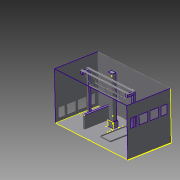
# Autodesk Inventor part: WTC
Saved by Autodesk Inventor 2013 (Build 170138000, 138)
## iProperties
Created: 2010-06-16
Part Number: WTC
Document SubType Name: Modeling
Designer: taylorm
Density: 1 g/cm^3
Material: Generic
Author: taylorm
Autodesk Inventor part; units mm, degrees
(part 1 of 2)
sketch "Sketch2" plane through (0, 0, 0) normal (0, 0, 1) x (1, 0, 0)
  line L0 (-3223.2861, 2012.2183) -> (3796.7139, 2012.2183)
  line L1 (3796.7139, 2012.2183) -> (3796.7139, -1587.7817)
  line L2 (3796.7139, -1587.7817) -> (-3223.2861, -1587.7817)
  line L3 (-3223.2861, -1587.7817) -> (-3223.2861, 2012.2183)
  point P0 (0, 0)
  dimension "d0" = 3600
  dimension "d1" = 7020
  constraints: 8 end point, 2 perpendicular, 1 horizontal, 1 parallel
  measures "d0" distance between parallel lines of L0 L2
  measures "d1" distance between parallel lines of L1 L3
ref_plane "Work Plane1" through (3796.7139, -1587.7817, 0) normal (0, 1, 0) x (-1, 0, 0)
sketch "Sketch4" plane through (3796.7139, -1587.7817, 0) normal (0, 1, 0) x (-1, 0, 0)
  line L0 (0, 0) -> (7020, 0) projected
  line L1 (0, 0) -> (0, -3820)
  line L2 (0, -3820) -> (7020, -3820)
  line L3 (7020, -3820) -> (7020, 0)
  point P0 (3796.7139, 0)
  dimension "d3" = 3820
  constraints: 6 end point, 3 perpendicular
  measures "d3" distance between parallel lines of L0 L2
ref_plane "Work Plane3" through (3796.7139, 2012.2183, 0) normal (0, 1, 0) x (-1, 0, 0)
sketch "Sketch5" plane through (3796.7139, 2012.2183, 0) normal (0, 1, 0) x (-1, 0, 0)
  line L0 (7020, -3820) -> (7020, 0) projected
  line L1 (0, -3820) -> (7020, -3820) projected
  line L2 (0, 0) -> (0, -3820) projected
  line L3 (7020, 0) -> (7020, -3820)
  line L4 (0, -3820) -> (0, 0)
  line L5 (0, -3820) -> (7020, -3820)
  point P0 (3796.7139, 0)
  constraints: 6 end point, 3 collinear
ref_plane "Work Plane4" through (3796.7139, 2012.2183, 0) normal (-1, 0, 0) x (0, 0, -1)
sketch "Sketch6" plane through (3796.7139, 2012.2183, 0) normal (-1, 0, 0) x (0, 0, -1)
  line L0 (0, 0) -> (3820, 0) projected
  line L1 (0, 3600) -> (3820, 3600) projected
  line L2 (0, 0) -> (0, 3600) projected
  line L3 (3820, 0) -> (3820, 3600)
  point P0 (0, 2012.2183)
  constraints: 2 end point, 1 parallel
ref_plane "Work Plane5" through (-3223.2861, -1587.7817, 0) normal (1, 0, 0) x (0, 0, -1)
sketch "Sketch7" plane through (-3223.2861, -1587.7817, 0) normal (1, 0, 0) x (0, 0, -1)
  line L0 (3820, 3600) -> (3820, 0) projected
  line L1 (3820, 0) -> (3820, 3600)
  point P0 (0, 1587.7817)
  constraints: 2 end point, 1 collinear
sketch "Sketch8" plane through (0, 0, 0) normal (0, 0, 1) x (1, 0, 0)
  line L0 (-663.2861, -147.7817) -> (-663.2861, -547.7817)
  line L1 (-663.2861, -547.7817) -> (-143.2861, -547.7817)
  line L2 (-143.2861, -547.7817) -> (-143.2861, -147.7817)
  line L3 (-143.2861, -147.7817) -> (-663.2861, -147.7817)
  line L4 (-3223.2861, -1587.7817) -> (-3223.2861, 2012.2183) projected
  line L5 (-3223.2861, 2012.2183) -> (3796.7139, 2012.2183) projected
  point P0 (0, 0)
  dimension "d4" = 2160
  dimension "d5" = 2560
  dimension "d6" = 400
  dimension "d7" = 520
  constraints: 8 end point, 2 parallel, 2 perpendicular, 1 vertical
  measures "d4" distance between parallel lines of L5 L3
  measures "d5" distance between parallel lines of L0 L4
  measures "d6" distance between parallel lines of L1 L3
  measures "d7" distance between parallel lines of L2 L0
ref_plane "Work Plane6" through (-663.2861, -147.7817, 0) normal (0, 1, 0) x (-1, 0, 0)
sketch "Sketch9" plane through (-663.2861, -147.7817, 0) normal (0, 1, 0) x (-1, 0, 0)
  line L0 (-520, 0) -> (0, 0) projected
  line L1 (0, 0) -> (0, -460)
  line L2 (0, -460) -> (-520, -460)
  line L3 (-520, -460) -> (-520, 0)
  point P0 (-663.2861, 0)
  dimension "d8" = 460
  constraints: 6 end point, 3 perpendicular
  measures "d8" distance between parallel lines of L0 L2
ref_plane "Work Plane7" through (-143.2861, -547.7817, 0) normal (0, 1, 0) x (-1, 0, 0)
sketch "Sketch10" plane through (-143.2861, -547.7817, 0) normal (0, 1, 0) x (-1, 0, 0)
  line L0 (520, -460) -> (0, -460) projected
  line L1 (0, -460) -> (0, 0) projected
  line L2 (520, 0) -> (520, -460) projected
  line L3 (520, 0) -> (0, 0) projected
  line L4 (0, 0) -> (0, -460)
  line L5 (520, -460) -> (0, -460)
  line L6 (520, -460) -> (520, 0)
  point P0 (-143.2861, 0)
  constraints: 6 end point, 2 perpendicular, 1 collinear
ref_plane "Work Plane8" through (-143.2861, -147.7817, 0) normal (1, 0, 0) x (0, 1, 0)
sketch "Sketch11" plane through (-143.2861, -147.7817, 0) normal (1, 0, 0) x (0, 1, 0)
  line L0 (0, -460) -> (0, 0) projected
  line L1 (-400, -460) -> (-400, 0) projected
  line L2 (-400, 0) -> (0, 0) projected
  line L3 (0, -460) -> (-400, -460)
  point P0 (147.7817, 0)
  constraints: 2 end point, 1 parallel
ref_plane "Work Plane9" through (-663.2861, -147.7817, -460) normal (1, 0, 0) x (0, 1, 0)
sketch "Sketch12" plane through (-663.2861, -147.7817, -460) normal (1, 0, 0) x (0, 1, 0)
  line L0 (0, 460) -> (-400, 460) projected
  line L1 (0, 460) -> (0, 0) projected
  line L2 (-400, 460) -> (-400, 0) projected
  line L3 (0, 0) -> (-400, 0)
  point P0 (147.7817, 460)
  constraints: 2 end point, 1 perpendicular
ref_plane "Work Plane10" through (-143.2861, -147.7817, -460) normal (0, 0, 1) x (1, 0, 0)
sketch "Sketch13" plane through (-143.2861, -147.7817, -460) normal (0, 0, 1) x (1, 0, 0)
  line L0 (-460, -55) -> (-60, -55)
  line L1 (-60, -55) -> (-60, -345)
  line L2 (-60, -345) -> (-460, -345)
  line L3 (-460, -345) -> (-460, -55)
  line L4 (-520, 0) -> (0, 0) projected
  line L5 (0, 0) -> (0, -400) projected
  line L6 (-520, -400) -> (0, -400) projected
  line L7 (-520, 0) -> (-520, -400) projected
  point P0 (143.2861, 147.7817)
  dimension "d9" = 60
  dimension "d10" = 60
  dimension "d11" = 55
  dimension "d12" = 55
  constraints: 8 end point, 2 parallel, 1 horizontal, 1 perpendicular
  measures "d9" distance between parallel lines of L7 L3
  measures "d10" distance between parallel lines of L5 L1
  measures "d11" distance between parallel lines of L4 L0
  measures "d12" distance between parallel lines of L6 L2
ref_plane "Work Plane11" through (-3223.2861, 2012.2183, -3820) normal (0, 0, 1) x (0, -1, 0)
sketch "Sketch14" plane through (-3223.2861, 2012.2183, -3820) normal (0, 0, 1) x (0, -1, 0)
  line L0 (2505, 2620) -> (2215, 2620) projected
  line L1 (2505, 3020) -> (2505, 2620) projected
  line L2 (2215, 3020) -> (2505, 3020) projected
  line L3 (2215, 2620) -> (2215, 3020) projected
  line L4 (2215, 2620) -> (2505, 2620)
  line L5 (2505, 3020) -> (2505, 2620)
  line L6 (2215, 3020) -> (2505, 3020)
  line L7 (2215, 2620) -> (2215, 3020)
  point P0 (2012.2183, 3223.2861)
  constraints: 8 end point, 3 perpendicular, 1 collinear
ref_plane "Work Plane12" through (-603.2861, -202.7817, -3820) normal (0, -1, 0) x (1, 0, 0)
sketch "Sketch15" plane through (-603.2861, -202.7817, -3820) normal (0, -1, 0) x (1, 0, 0)
  line L0 (0, 0) -> (400, 0) projected
  line L1 (0, 3360) -> (400, 3360) projected
  line L2 (0, 0) -> (0, 3360)
  line L3 (400, 3360) -> (400, 0)
  point P0 (603.2861, 3820)
  constraints: 4 end point, 1 parallel, 1 perpendicular
ref_plane "Work Plane14" through (-203.2861, -492.7817, -460) normal (0, 1, 0) x (0, 0, -1)
sketch "Sketch16" plane through (-203.2861, -492.7817, -460) normal (0, 1, 0) x (0, 0, -1)
  line L0 (3360, 0) -> (3360, 400) projected
  line L1 (0, 0) -> (0, 400) projected
  line L2 (0, 0) -> (3360, 0) projected
  line L3 (3360, 400) -> (0, 400) projected
  line L4 (3360, 0) -> (0, 0)
  line L5 (0, 400) -> (3360, 400)
  point P0 (-460, -203.2861)
  constraints: 4 end point, 2 collinear
sketch "Sketch17" plane through (0, 0, 0) normal (0, 0, 1) x (1, 0, 0)
  line L0 (-3223.2861, -1587.7817) -> (-3223.2861, 2012.2183) projected
  line L1 (-3223.2861, 2012.2183) -> (3796.7139, 2012.2183) projected
  line L2 (3796.7139, -1587.7817) -> (-3223.2861, -1587.7817) projected
  line L3 (3796.7139, 2012.2183) -> (3796.7139, -1587.7817) projected
  line L4 (-1423.2861, -807.7817) -> (-1423.2861, -781.363)
  line L5 (-1423.2861, -781.363) -> (-1423.2861, 1242.2183)
  line L6 (-1423.2861, 1242.2183) -> (-1273.2861, 1242.2183)
  line L7 (-1273.2861, 1242.2183) -> (-1273.2861, -807.7817)
  line L8 (-1273.2861, -807.7817) -> (-1423.2861, -807.7817)
  point P0 (0, 0)
  dimension "d13" = 770
  dimension "d14" = 2050
  dimension "d15" = 150
  dimension "d16" = 1800
  constraints: 10 end point, 3 perpendicular, 1 collinear, 1 parallel
  measures "d13" distance between parallel lines of L1 L6
  measures "d14" distance between parallel lines of L8 L6
  measures "d15" distance between parallel lines of L7 L5
  measures "d16" distance between parallel lines of L0 L5
ref_plane "Work Plane15" through (-1273.2861, 1242.2183, 0) normal (0, 1, 0) x (-1, 0, 0)
sketch "Sketch18" plane through (-1273.2861, 1242.2183, 0) normal (0, 1, 0) x (-1, 0, 0)
  line L0 (150, 0) -> (0, 0) projected
  line L1 (0, 0) -> (0, -1000)
  line L2 (0, -1000) -> (150, -1000)
  line L3 (150, -1000) -> (150, 0)
  point P0 (-1273.2861, 0)
  dimension "d17" = 1000
  constraints: 6 end point, 2 perpendicular, 1 parallel
  measures "d17" distance between parallel lines of L0 L2
ref_plane "Work Plane16" through (-1273.2861, -807.7817, 0) normal (0, 1, 0) x (-1, 0, 0)
sketch "Sketch19" plane through (-1273.2861, -807.7817, 0) normal (0, 1, 0) x (-1, 0, 0)
  line L0 (0, 0) -> (150, 0) projected
  line L1 (150, -1000) -> (150, 0) projected
  line L2 (0, 0) -> (0, -1000) projected
  line L3 (0, -1000) -> (150, -1000) projected
  line L4 (0, 0) -> (0, -1000)
  line L5 (150, -1000) -> (0, -1000)
  line L6 (150, -1000) -> (150, 0)
  point P0 (-1273.2861, 0)
  constraints: 6 end point, 2 collinear, 1 perpendicular
ref_plane "Work Plane17" through (-1273.2861, 1242.2183, -1000) normal (0, 0, 1) x (1, 0, 0)
sketch "Sketch20" plane through (-1273.2861, 1242.2183, -1000) normal (0, 0, 1) x (1, 0, 0)
  line L0 (0, 0) -> (-150, 0) projected
  line L1 (-150, -2050) -> (0, -2050) projected
  line L2 (0, 0) -> (0, -2050)
  line L3 (-150, 0) -> (-150, -2050)
  point P0 (1273.2861, -1242.2183)
  constraints: 4 end point, 1 parallel, 1 perpendicular
sketch "Sketch21" plane through (0, 0, 0) normal (0, 0, 1) x (1, 0, 0)
  line L0 (-3223.2861, -1587.7817) -> (-3223.2861, 2012.2183) projected
  line L1 (-3223.2861, 2012.2183) -> (3796.7139, 2012.2183) projected
  line L2 (3796.7139, -1587.7817) -> (-3223.2861, -1587.7817) projected
  line L3 (-1963.2861, 252.2183) -> (-1963.2861, 417.2183)
  line L4 (-1963.2861, 417.2183) -> (-1798.2861, 417.2183)
  line L5 (-1798.2861, 417.2183) -> (-1798.2861, 252.2183)
  line L6 (-1798.2861, 252.2183) -> (-1963.2861, 252.2183)
  point P0 (0, 0)
  dimension "d18" = 1840
  dimension "d19" = 165
  dimension "d20" = 165
  dimension "d21" = 1260
  constraints: 8 end point, 2 parallel, 2 perpendicular
  measures "d18" distance from line of L3.start L2
  measures "d19" distance of L3.start L3.end
  measures "d20" distance of L4.end L3.end
  measures "d21" distance between parallel lines of L0 L3
ref_plane "Work Plane18" through (-1963.2861, 417.2183, 0) normal (1, 0, 0) x (0, 1, 0)
sketch "Sketch22" plane through (-1963.2861, 417.2183, 0) normal (1, 0, 0) x (0, 1, 0)
  line L0 (-165, 0) -> (0, 0) projected
  line L1 (0, 0) -> (0, -3555)
  line L2 (0, -3555) -> (-165, -3555)
  line L3 (-165, -3555) -> (-165, 0)
  point P0 (-417.2183, 0)
  dimension "d22" = 3555
  constraints: 6 end point, 2 perpendicular, 1 parallel
  measures "d22" distance of L0.end L1.end
ref_plane "Work Plane19" through (-1798.2861, 417.2183, 0) normal (1, 0, 0) x (0, 1, 0)
sketch "Sketch23" plane through (-1798.2861, 417.2183, 0) normal (1, 0, 0) x (0, 1, 0)
  line L0 (0, 0) -> (0, -3555) projected
  line L1 (-165, -3555) -> (-165, 0) projected
  line L2 (0, -3555) -> (-165, -3555) projected
  line L3 (0, 0) -> (0, -3555)
  line L4 (0, -3555) -> (-165, -3555)
  line L5 (-165, -3555) -> (-165, 0)
  point P0 (-417.2183, 0)
  constraints: 6 end point, 2 collinear, 1 perpendicular
ref_plane "Work Plane20" through (-1963.2861, 417.2183, -3555) normal (0, 0, 1) x (1, 0, 0)
sketch "Sketch24" plane through (-1963.2861, 417.2183, -3555) normal (0, 0, 1) x (1, 0, 0)
  line L0 (0, 0) -> (0, -165) projected
  line L1 (165, -165) -> (0, -165) projected
  line L2 (165, 0) -> (165, -165) projected
  line L3 (0, 0) -> (165, 0) projected
  line L4 (0, -165) -> (165, -165)
  line L5 (165, 0) -> (0, 0)
  line L6 (0, -165) -> (165, -165)
  line L7 (165, -165) -> (165, 495)
  line L8 (165, 495) -> (0, 495)
  line L9 (0, 495) -> (0, -165)
  point P0 (1963.2861, -417.2183)
  dimension "d23" = 660
  constraints: 12 end point, 3 collinear, 2 perpendicular, 1 parallel
  measures "d23" distance between parallel lines of L8 L6
ref_plane "Work Plane21" through (-1798.2861, 912.2183, -3555) normal (1, 0, 0) x (0, 1, 0)
sketch "Sketch25" plane through (-1798.2861, 912.2183, -3555) normal (1, 0, 0) x (0, 1, 0)
  line L0 (-660, 0) -> (0, 0) projected
  line L1 (0, 0) -> (0, -165)
  line L2 (0, -165) -> (-660, -165)
  line L3 (-660, -165) -> (-660, 0)
  point P0 (-912.2183, 3555)
  dimension "d24" = 165
  constraints: 6 end point, 2 perpendicular, 1 parallel
  measures "d24" distance between parallel lines of L0 L2
ref_plane "Work Plane22" through (-1963.2861, 252.2183, -3555) normal (1, 0, 0) x (0, 1, 0)
sketch "Sketch26" plane through (-1963.2861, 252.2183, -3555) normal (1, 0, 0) x (0, 1, 0)
  line L0 (660, -165) -> (0, -165) projected
  line L1 (660, 0) -> (660, -165) projected
  line L2 (0, -165) -> (0, 0) projected
  line L3 (0, 0) -> (0, -165)
  line L4 (0, -165) -> (660, -165)
  line L5 (660, -165) -> (660, 0)
  point P0 (-252.2183, 3555)
  constraints: 6 end point, 2 collinear, 1 perpendicular
ref_plane "Work Plane23" through (-1798.2861, 912.2183, -3720) normal (0, 0, 1) x (1, 0, 0)
sketch "Sketch27" plane through (-1798.2861, 912.2183, -3720) normal (0, 0, 1) x (1, 0, 0)
  line L0 (0, 0) -> (0, -660) projected
  line L1 (-165, 0) -> (-165, -660) projected
  line L2 (0, 0) -> (-165, 0)
  line L3 (0, -660) -> (-165, -660)
  point P0 (1798.2861, -912.2183)
  constraints: 4 end point, 1 parallel, 1 perpendicular
sketch "Sketch28" plane through (0, 0, 0) normal (0, 0, 1) x (1, 0, 0)
  line L0 (2381.7139, 417.2183) -> (2381.7139, 252.2183)
  line L1 (2381.7139, 252.2183) -> (2546.7139, 252.2183)
  line L2 (2546.7139, 252.2183) -> (2546.7139, 417.2183)
  line L3 (2546.7139, 417.2183) -> (2381.7139, 417.2183)
  line L4 (3796.7139, -1587.7817) -> (-3223.2861, -1587.7817) projected
  line L5 (3796.7139, 2012.2183) -> (3796.7139, -1587.7817) projected
  point P0 (0, 0)
  dimension "d25" = 1840
  dimension "d26" = 1250
  dimension "d27" = 165
  dimension "d28" = 165
  constraints: 8 end point, 2 parallel, 1 perpendicular, 1 vertical
  measures "d25" distance between parallel lines of L4 L1
  measures "d26" distance between parallel lines of L5 L2
  measures "d27" distance between parallel lines of L2 L0
  measures "d28" distance of L1.end L2.end
ref_plane "Work Plane24" through (2546.7139, 417.2183, 0) normal (1, 0, 0) x (0, 1, 0)
sketch "Sketch29" plane through (2546.7139, 417.2183, 0) normal (1, 0, 0) x (0, 1, 0)
  line L0 (-165, -3555) -> (-165, 0) projected
  line L1 (-165, -3555) -> (-165, 0) projected
  line L2 (0, 0) -> (0, -3555) projected
  line L3 (0, -3555) -> (-165, -3555) projected
  line L4 (-165, -3555) -> (495, -3555) projected
  line L5 (0, 0) -> (0, -3555)
  line L6 (0, -3555) -> (-165, -3555)
  line L7 (-165, -3555) -> (-165, 0)
  line L8 (-165, -3555) -> (495, -3555)
  line L9 (495, -3555) -> (495, -3720) projected
  line L10 (495, -3720) -> (-165, -3720) projected
  line L11 (-165, -3720) -> (-165, -3555) projected
  line L12 (495, -3555) -> (495, -3720)
  line L13 (-165, -3720) -> (-165, -3555)
  line L14 (495, -3720) -> (-165, -3720)
  point P0 (-417.2183, 0)
  constraints: 14 end point, 6 equal length, 1 perpendicular
ref_plane "Work Plane25" through (2381.7139, 417.2183, 0) normal (1, 0, 0) x (0, 1, 0)
sketch "Sketch30" plane through (2381.7139, 417.2183, 0) normal (1, 0, 0) x (0, 1, 0)
  line L0 (0, 0) -> (0, -3555) projected
  line L1 (-165, -3555) -> (-165, 0) projected
  line L2 (-165, -3555) -> (495, -3555) projected
  line L3 (495, -3720) -> (-165, -3720) projected
  line L4 (495, -3555) -> (495, -3720) projected
  line L5 (-165, -3720) -> (-165, -3555) projected
  line L6 (0, -3555) -> (-165, -3555) projected
  line L7 (495, -3555) -> (495, -3720)
  line L8 (-165, -3720) -> (495, -3720)
  line L9 (495, -3555) -> (-165, -3555)
  line L10 (-165, -3555) -> (-165, -3720)
  line L11 (-165, -3555) -> (0, -3555)
  line L12 (0, -3555) -> (0, 0)
  line L13 (-165, 0) -> (-165, -3555)
  point P0 (-417.2183, 0)
  constraints: 14 end point, 5 collinear, 1 parallel, 1 perpendicular
ref_plane "Work Plane26" through (2381.7139, 912.2183, -3720) normal (0, 1, 0) x (0, 0, 1)
sketch "Sketch31" plane through (2381.7139, 912.2183, -3720) normal (0, 1, 0) x (0, 0, 1)
  line L0 (165, 165) -> (0, 165) projected
  line L1 (165, 0) -> (0, 0) projected
  line L2 (165, 0) -> (165, 165)
  line L3 (0, 165) -> (0, 0)
  point P0 (3720, -2381.7139)
  constraints: 4 end point, 1 parallel, 1 perpendicular
ref_plane "Work Plane27" through (2546.7139, 252.2183, -3720) normal (0, -1, 0) x (0, 0, 1)
sketch "Sketch32" plane through (2546.7139, 252.2183, -3720) normal (0, -1, 0) x (0, 0, 1)
  line L0 (0, 0) -> (0, 165) projected
  line L1 (165, 165) -> (165, 0) projected
  line L2 (0, 0) -> (0, 165)
  line L3 (165, 165) -> (165, 0)
  point P0 (3720, 2546.7139)
  constraints: 4 end point, 2 equal length
ref_plane "Work Plane28" through (2546.7139, 417.2183, -3555) normal (0, 1, 0) x (-1, 0, 0)
sketch "Sketch33" plane through (2546.7139, 417.2183, -3555) normal (0, 1, 0) x (-1, 0, 0)
  line L0 (165, 0) -> (0, 0) projected
  line L1 (165, 0) -> (0, 0)
  point P0 (2546.7139, 3555)
  constraints: 2 end point, 1 collinear
extrude "Extrusion1" add sketch "Sketch9" against normal up to surface (400 mm away)
extrude "Extrusion2" add sketch "Sketch15" along normal up to surface (290 mm away)
extrude "Extrusion3" add sketch "Sketch18" against normal up to surface (2050 mm away) separate body
extrude "Extrusion4" add sketch "Sketch31" against normal up to surface (660 mm away) separate body
extrude "Extrusion5" add sketch "Sketch22" along normal up to surface (165 mm away) separate body
extrude "Extrusion6" add sketch "Sketch27" along normal up to surface (165 mm away) separate body
extrude "Extrusion7" add sketch "Sketch17" along normal blind 25 separate body
extrude "Extrusion8" add sketch "Sketch4" along normal blind 25 separate body
ref_plane "Work Plane29" through (-3223.2861, 2012.2183, -3820) normal (0, 1, 0) x (-1, 0, 0)
extrude "Extrusion10" add sketch "Sketch28" against normal up to surface (3555 mm away) separate body
sketch "Sketch34" plane through (-3223.2861, 2012.2183, -3820) normal (0, 1, 0) x (-1, 0, 0)
  line L0 (-7020, 0) -> (0, 0) projected
  line L1 (0, 0) -> (0, 3820) projected
  line L2 (-7020, 3820) -> (-7020, 0) projected
  line L3 (0, 3820) -> (-7020, 3820) projected
  line L4 (0, 0) -> (-7020, 0)
  line L5 (-7020, 3820) -> (-7020, 0)
  line L6 (-7020, 3820) -> (0, 3820)
  line L7 (0, 3820) -> (0, 0)
  point P0 (-3223.2861, 3820)
  constraints: 8 end point, 4 collinear
extrude "Extrusion9" [suppressed]
ref_plane "Work Plane30" through (3796.7139, 2012.2183, -3820) normal (1, 0, 0) x (0, 1, 0)
sketch "Sketch35" plane through (3796.7139, 2012.2183, -3820) normal (1, 0, 0) x (0, 1, 0)
  line L0 (0, 0) -> (-3600, 0) projected
  line L1 (0, 3820) -> (0, 0) projected
  line L2 (0, 3845) -> (-3600, 3845) projected
  line L3 (-3600, 3820) -> (-3600, 0) projected
  line L4 (-300, 1000) -> (-800, 1000)
  line L5 (-800, 1000) -> (-800, 1700)
  line L6 (-800, 1700) -> (-300, 1700)
  line L7 (-300, 1700) -> (-300, 1000)
  line L8 (-1000, 1000) -> (-1000, 1700)
  line L9 (-1000, 1700) -> (-1700, 1700)
  line L10 (-1700, 1700) -> (-1700, 1000)
  line L11 (-1700, 1000) -> (-1000, 1000)
  line L12 (-1900, 1000) -> (-1900, 1700)
  line L13 (-1900, 1700) -> (-2600, 1700)
  line L14 (-2600, 1700) -> (-2600, 1000)
  line L15 (-2600, 1000) -> (-1900, 1000)
  line L16 (-2800, 1000) -> (-2800, 1700)
  line L17 (-2800, 1700) -> (-3300, 1700)
  line L18 (-3300, 1700) -> (-3300, 1000)
  line L19 (-3300, 1000) -> (-2800, 1000)
  line L20 (-300, 1000) -> (-800, 1000)
  line L21 (-800, 1700) -> (-800, 1000)
  line L22 (-800, 1000) -> (-300, 1000)
  line L23 (-1000, 1000) -> (-1700, 1000)
  line L24 (-1700, 1000) -> (-1700, 1700)
  line L25 (-1700, 1700) -> (-1000, 1700)
  line L26 (-1000, 1700) -> (-1000, 1000)
  line L27 (-1900, 1000) -> (-2600, 1000)
  line L28 (-2600, 1000) -> (-2600, 1700)
  line L29 (-2600, 1700) -> (-1900, 1700)
  line L30 (-1900, 1700) -> (-1900, 1000)
  line L31 (-2800, 1000) -> (-3300, 1000)
  line L32 (-3300, 1000) -> (-3300, 1700)
  line L33 (-3300, 1700) -> (-2800, 1700)
  line L34 (-2800, 1700) -> (-2800, 1000)
  point P0 (-2012.2183, 3820)
  dimension "d49" = 700
  dimension "d50" = 700
  dimension "d51" = 700
  dimension "d52" = 700
  dimension "d53" = 500
  dimension "d54" = 700
  dimension "d55" = 700
  dimension "d56" = 500
  dimension "d57" = 1000
  dimension "d58" = 300
  dimension "d59" = 300
  dimension "d60" = 200
  dimension "d61" = 200
  dimension "d62" = 200
  constraints: 62 end point, 15 perpendicular, 10 parallel, 9 collinear
  measures "d49" distance between parallel lines of L6 L4
  measures "d50" distance between parallel lines of L9 L11
  measures "d51" distance between parallel lines of L13 L15
  measures "d52" distance between parallel lines of L17 L19
  measures "d53" distance between parallel lines of L5 L7
  measures "d54" distance between parallel lines of L10 L8
  measures "d55" distance between parallel lines of L14 L12
  measures "d56" distance between parallel lines of L18 L16
  measures "d57" distance between parallel lines of L4 L0
  measures "d58" distance between parallel lines of L7 L1
  measures "d59" distance between parallel lines of L3 L18
  measures "d60" distance between parallel lines of L8 L5
  measures "d61" distance between parallel lines of L16 L14
  measures "d62" distance between parallel lines of L12 L10
ref_plane "Work Plane32" through (3796.7139, 2012.2183, -3820) normal (1, 0, 0) x (0, 0, 1)
sketch "Sketch37" plane through (3796.7139, 2012.2183, -3820) normal (1, 0, 0) x (0, 0, 1)
  line L0 (0, 0) -> (0, 3600) projected
  line L1 (0, 0) -> (3820, 0) projected
  line L2 (3820, 0) -> (3820, 3600) projected
  line L3 (3845, 0) -> (3845, 3600) projected
  line L4 (3820, 3600) -> (0, 3600) projected
  line L5 (1000, 300) -> (1000, 800) projected
  line L6 (1700, 300) -> (1000, 300) projected
  line L7 (1700, 800) -> (1700, 300) projected
  line L8 (1000, 800) -> (1700, 800) projected
  line L9 (1700, 1000) -> (1000, 1000) projected
  line L10 (1000, 1700) -> (1000, 1000) projected
  line L11 (1700, 1000) -> (1700, 1700) projected
  line L12 (1700, 1700) -> (1000, 1700) projected
  line L13 (1000, 2600) -> (1000, 1900) projected
  line L14 (1000, 1900) -> (1700, 1900) projected
  line L15 (1700, 1900) -> (1700, 2600) projected
  line L16 (1700, 2600) -> (1000, 2600) projected
  line L17 (1700, 2800) -> (1000, 2800) projected
  line L18 (1000, 3300) -> (1000, 2800) projected
  line L19 (1700, 3300) -> (1000, 3300) projected
  line L20 (1700, 2800) -> (1700, 3300) projected
  line L21 (1000, 300) -> (1000, 800)
  line L22 (1000, 800) -> (1700, 800)
  line L23 (1700, 800) -> (1700, 300)
  line L24 (1700, 300) -> (1000, 300)
  line L25 (0, 0) -> (0, 3600)
  line L26 (0, 3600) -> (3845, 3600)
  line L27 (3845, 3600) -> (3845, 0)
  line L28 (3845, 0) -> (0, 0)
  line L29 (1000, 1000) -> (1000, 1700)
  line L30 (1000, 1700) -> (1700, 1700)
  line L31 (1700, 1700) -> (1700, 1000)
  line L32 (1700, 1000) -> (1000, 1000)
  line L33 (1000, 1900) -> (1000, 2600)
  line L34 (1000, 2600) -> (1700, 2600)
  line L35 (1700, 2600) -> (1700, 1900)
  line L36 (1700, 1900) -> (1000, 1900)
  line L37 (1000, 2800) -> (1000, 3300)
  line L38 (1000, 3300) -> (1700, 3300)
  line L39 (1700, 3300) -> (1700, 2800)
  line L40 (1700, 2800) -> (1000, 2800)
  point P0 (3820, 2012.2183)
  constraints: 40 end point, 15 perpendicular, 5 equal length
extrude "Extrusion12" add sketch "Sketch37" against normal blind 25 separate body contours L0 L4 L2 L1
ref_plane "Work Plane33" through (-3223.2861, -1587.7817, -3820) normal (1, 0, 0) x (0, 1, 0)
sketch "Sketch38" plane through (-3223.2861, -1587.7817, -3820) normal (1, 0, 0) x (0, 1, 0)
  line L0 (0, 3820) -> (0, 0) projected
  line L1 (3600, 0) -> (0, 0) projected
  line L2 (3600, 0) -> (3600, 3820) projected
  line L3 (0, 3845) -> (3600, 3845) projected
  line L4 (0, 3845) -> (3600, 3845)
  line L5 (3600, 3845) -> (3600, 0)
  line L6 (3600, 0) -> (0, 0)
  line L7 (0, 0) -> (0, 3845)
  line L8 (300, 3545) -> (800, 3545)
  line L9 (800, 3545) -> (800, 2845)
  line L10 (800, 2845) -> (300, 2845)
  line L11 (300, 2845) -> (300, 3545)
  line L12 (1000, 3545) -> (1000, 2845)
  line L13 (1000, 2845) -> (1700, 2845)
  line L14 (1700, 2845) -> (1700, 3545)
  line L15 (1700, 3545) -> (1000, 3545)
  line L16 (1900, 3545) -> (1900, 2845)
  line L17 (1900, 2845) -> (2600, 2845)
  line L18 (2600, 2845) -> (2600, 3545)
  line L19 (2600, 3545) -> (1900, 3545)
  line L20 (2800, 3545) -> (2800, 2845)
  line L21 (2800, 2845) -> (3300, 2845)
  line L22 (3300, 2845) -> (3300, 3545)
  line L23 (3300, 3545) -> (2800, 3545)
  point P0 (1587.7817, 3820)
  dimension "d67" = 300
  dimension "d68" = 700
  dimension "d69" = 500
  dimension "d70" = 700
  dimension "d71" = 700
  dimension "d72" = 500
  dimension "d73" = 300
  dimension "d74" = 300
  dimension "d75" = 200
  dimension "d76" = 200
  dimension "d77" = 200
  constraints: 40 end point, 11 perpendicular, 9 equal length, 6 collinear
  measures "d67" distance between parallel lines of L3 L8
  measures "d68" distance between parallel lines of L8 L10
  measures "d69" distance between parallel lines of L9 L11
  measures "d70" distance between parallel lines of L14 L12
  measures "d71" distance between parallel lines of L18 L16
  measures "d72" distance between parallel lines of L22 L20
  measures "d73" distance between parallel lines of L0 L11
  measures "d74" distance between parallel lines of L2 L22
  measures "d75" distance between parallel lines of L9 L12
  measures "d76" distance between parallel lines of L14 L16
  measures "d77" distance between parallel lines of L18 L20
extrude "Extrusion13" add sketch "Sketch38" against normal blind 25 separate body
ref_plane "Work Plane34" through (-3223.2861, 2024.7183, -3820) normal (0, 0, -1) x (0.9999984, 0.0017806, 0)
sketch "Sketch39" plane through (-3223.2861, 2024.7183, -3820) normal (0, 0, -1) x (0.9999984, 0.0017806, 0)
  line L0 (-31.4325, 3612.4498) -> (-25.0222, 12.4555) projected
  line L1 (0.0223, -12.5) -> (7020.0111, 0) projected
  line L2 (7019.9666, 25) -> (7013.5564, 3624.9943) projected
  line L3 (-6.4325, 3612.4943) -> (7013.5564, 3624.9943) projected
  line L4 (0.0223, -12.5) -> (-6.4325, 3612.4943)
  line L5 (-6.4325, 3612.4943) -> (7013.5564, 3624.9943)
  line L6 (7013.5564, 3624.9943) -> (7019.9666, 25)
  line L7 (7019.9666, 25) -> (0.0223, -12.5)
  point P0 (3219.6757, 2030.4546)
  constraints: 8 end point, 3 perpendicular
extrude "Extrusion14" [suppressed]
ref_plane "Work Plane35" through (2546.7139, 912.2183, -3720) normal (1, 0, 0) x (0, 1, 0)
sketch "Sketch40" plane through (2546.7139, 912.2183, -3720) normal (1, 0, 0) x (0, 1, 0)
  line L0 (-69.6, 0) -> (-76, 0)
  line L1 (-76, 0) -> (-76, -76)
  line L2 (-76, -76) -> (0, -76)
  line L3 (0, -76) -> (0, -69.6)
  line L4 (0, -69.6) -> (-69.6, -69.6)
  line L5 (-69.6, -69.6) -> (-69.6, 0)
  line L6 (-101.6, 0) -> (-101.6, -76)
  line L7 (-101.6, -76) -> (-177.6, -76)
  line L8 (-177.6, -76) -> (-177.6, -69.6)
  line L9 (-177.6, -69.6) -> (-108, -69.6)
  line L10 (-108, -69.6) -> (-108, 0)
  line L11 (-108, 0) -> (-101.6, 0)
  line L12 (0, 0) -> (-660, 0) projected
  line L13 (0, 165) -> (0, 0) projected
  point P0 (-912.2183, 3720)
  dimension "d96" = 25.6
  dimension "d97" = 6.4
  dimension "d98" = 6.4
  dimension "d99" = 76
  dimension "d100" = 6.4
  dimension "d101" = 76
  dimension "d102" = 76
  constraints: 24 end point, 9 parallel, 5 collinear, 2 perpendicular, 1 horizontal
  measures "d96" distance between parallel lines of L6 L1
  measures "d97" distance between parallel lines of L5 L1
  measures "d98" distance between parallel lines of L4 L2
  measures "d99" distance between parallel lines of L0 L2
  measures "d100" distance between parallel lines of L10 L6
  measures "d101" distance of L1.end L2.end
  measures "d102" distance of L6.end L7.end
extrude "Extrusion15" add sketch "Sketch40" against normal blind 4600 separate body
sketch "Sketch41" plane through (2546.7139, 912.2183, -3720) normal (1, 0, 0) x (0, 1, 0)
  line L0 (0, 0) -> (-660, 0) projected
  line L1 (-660, 0) -> (-660, 165) projected
  line L2 (-660, -76) -> (-660, -69.6)
  line L3 (-660, -69.6) -> (-590.4, -69.6)
  line L4 (-590.4, -69.6) -> (-590.4, 0)
  line L5 (-584, 0) -> (-584, -76)
  line L6 (-584, -76) -> (-660, -76)
  line L7 (-558.4, -76) -> (-558.4, 0)
  line L8 (-552, 0) -> (-552, -69.6)
  line L9 (-552, -69.6) -> (-482.4, -69.6)
  line L10 (-482.4, -69.6) -> (-482.4, -76)
  line L11 (-482.4, -76) -> (-558.4, -76)
  point P0 (-912.2183, 3720)
  dimension "d105" = 25.6
  dimension "d106" = 6.4
  dimension "d107" = 6.4
  dimension "d108" = 6.4
  dimension "d109" = 6.4
  dimension "d110" = 76
  dimension "d111" = 76
  dimension "d112" = 76
  constraints: 20 end point, 5 parallel, 4 perpendicular, 4 point on line, 2 collinear
  measures "d105" distance between parallel lines of L5 L7
  measures "d106" distance between parallel lines of L7 L8
  measures "d107" distance between parallel lines of L4 L5
  measures "d108" distance between parallel lines of L11 L9
  measures "d109" distance between parallel lines of L6 L3
  measures "d110" distance between parallel lines of L0 L11
  measures "d111" distance between parallel lines of L7 L10
  measures "d112" distance between parallel lines of L2 L5
extrude "Extrusion16" add sketch "Sketch41" against normal blind 4600 separate body
sketch "Sketch42" plane through (0, 0, 0) normal (0, 1, 0) x (-1, 0, 0)
  line L0 (-2546.7139, -3555) -> (-2546.7139, -3720) projected
  point P0 (0, 0)
  point P1 (-1746.7139, -2598.7334)
  dimension "d115" = 800
  measures "d115" distance from line of L0 point (-1746.714, -2598.733)
ref_plane "Work Plane36" through (1746.7139, 0, -2598.7334) normal (1, 0, 0) x (0, 1, 0)
sketch "Sketch43" plane through (1746.7139, 0, -2598.7334) normal (1, 0, 0) x (0, 1, 0)
  line L0 (842.6183, -1190.8666) -> (842.6183, -1121.2666) projected
  line L1 (836.2183, -1121.2666) -> (836.2183, -1197.2666) projected
  line L2 (810.6183, -1121.2666) -> (810.6183, -1197.2666) projected
  line L3 (804.2183, -1190.8666) -> (804.2183, -1121.2666) projected
  line L4 (836.2183, -1197.2666) -> (912.2183, -1197.2666) projected
  line L5 (912.2183, -1190.8666) -> (842.6183, -1190.8666) projected
  line L6 (734.6183, -1190.8666) -> (804.2183, -1190.8666) projected
  line L7 (810.6183, -1197.2666) -> (734.6183, -1197.2666) projected
  line L8 (429.8183, -1190.8666) -> (360.2183, -1190.8666) projected
  line L9 (353.8183, -1197.2666) -> (429.8183, -1197.2666) projected
  line L10 (360.2183, -1190.8666) -> (360.2183, -1121.2666) projected
  line L11 (353.8183, -1121.2666) -> (353.8183, -1197.2666) projected
  line L12 (252.2183, -1197.2666) -> (328.2183, -1197.2666) projected
  line L13 (321.8183, -1190.8666) -> (252.2183, -1190.8666) projected
  line L14 (321.8183, -1121.2666) -> (321.8183, -1190.8666) projected
  line L15 (328.2183, -1197.2666) -> (328.2183, -1121.2666) projected
  line L16 (836.2183, -461.2666) -> (836.2183, -397.2666)
  line L17 (836.2183, -397.2666) -> (900.2183, -397.2666)
  line L18 (900.2183, -397.2666) -> (900.2183, -403.6666)
  line L19 (900.2183, -403.6666) -> (842.6183, -403.6666)
  line L20 (842.6183, -403.6666) -> (842.6183, -461.2666)
  line L21 (842.6183, -461.2666) -> (836.2183, -461.2666)
  line L22 (810.6183, -461.2666) -> (810.6183, -397.2666)
  line L23 (810.6183, -397.2666) -> (746.6183, -397.2666)
  line L24 (746.6183, -397.2666) -> (746.6183, -403.6666)
  line L25 (746.6183, -403.6666) -> (804.2183, -403.6666)
  line L26 (804.2183, -403.6666) -> (804.2183, -461.2666)
  line L27 (804.2183, -461.2666) -> (810.6183, -461.2666)
  line L28 (582.1183, -366.7886) -> (582.1183, -833.5683)
  point P0 (0, 2598.7334)
  dimension "d116" = 6.4
  dimension "d117" = 6.4
  dimension "d118" = 6.4
  dimension "d119" = 6.4
  dimension "d120" = 64
  dimension "d121" = 64
  dimension "d122" = 64
  dimension "d123" = 25.6
  dimension "d124" = 800
  dimension "d125" = 228.5
  constraints: 26 end point, 9 parallel, 4 perpendicular, 3 collinear
  measures "d116" distance between parallel lines of L16 L20
  measures "d117" distance between parallel lines of L26 L22
  measures "d118" distance between parallel lines of L19 L17
  measures "d119" distance between parallel lines of L25 L23
  measures "d120" distance between parallel lines of L21 L17
  measures "d121" distance between parallel lines of L18 L16
  measures "d122" distance between parallel lines of L24 L22
  measures "d123" distance between parallel lines of L22 L16
  measures "d124" distance between parallel lines of L4 L17
  measures "d125" distance between parallel lines of L28 L22
extrude "Extrusion17" add sketch "Sketch43" against normal blind 3000 separate body
sketch "Sketch44" plane through (1746.7139, 0, -2598.7334) normal (1, 0, 0) x (0, 1, 0)
  line L0 (353.8183, -1121.2666) -> (353.8183, -1197.2666) projected
  line L1 (360.2183, -1190.8666) -> (360.2183, -1121.2666) projected
  line L2 (328.2183, -1197.2666) -> (328.2183, -1121.2666) projected
  line L3 (321.8183, -1121.2666) -> (321.8183, -1190.8666) projected
  line L4 (252.2183, -1197.2666) -> (328.2183, -1197.2666) projected
  line L5 (353.8183, -1197.2666) -> (429.8183, -1197.2666) projected
  line L6 (810.6183, -397.2666) -> (746.6183, -397.2666) projected
  line L7 (836.2183, -397.2666) -> (900.2183, -397.2666) projected
  line L8 (353.8183, -397.2666) -> (402.4631, -397.2666)
  line L9 (402.4631, -397.2666) -> (402.4631, -403.6666)
  line L10 (402.4631, -403.6666) -> (360.2183, -403.6666)
  line L11 (360.2183, -403.6666) -> (360.2183, -461.2666)
  line L12 (360.2183, -461.2666) -> (353.8183, -461.2666)
  line L13 (353.8183, -461.2666) -> (353.8183, -397.2666)
  line L14 (328.2183, -397.2666) -> (328.2183, -461.2666)
  line L15 (328.2183, -461.2666) -> (321.8183, -461.2666)
  line L16 (321.8183, -461.2666) -> (321.8183, -403.6666)
  line L17 (321.8183, -403.6666) -> (283.0913, -403.6666)
  line L18 (283.0913, -403.6666) -> (283.0913, -397.2666)
  line L19 (283.0913, -397.2666) -> (328.2183, -397.2666)
  point P0 (0, 2598.7334)
  dimension "d128" = 6.4
  dimension "d129" = 6.4
  dimension "d130" = 64
  dimension "d131" = 64
  dimension "d132" = 25.6
  dimension "d133" = 6.4
  dimension "d134" = 6.4
  dimension "d135" = 800
  constraints: 24 end point, 9 parallel, 3 collinear, 2 perpendicular
  measures "d128" distance between parallel lines of L8 L10
  measures "d129" distance between parallel lines of L19 L17
  measures "d130" distance between parallel lines of L8 L12
  measures "d131" distance between parallel lines of L19 L15
  measures "d132" distance between parallel lines of L14 L13
  measures "d133" distance between parallel lines of L13 L11
  measures "d134" distance between parallel lines of L16 L14
  measures "d135" distance between parallel lines of L5 L8
extrude "Extrusion18" add sketch "Sketch44" against normal blind 3000 separate body
sketch "Sketch45" plane through (1746.7139, 0, -2598.7334) normal (1, 0, 0) x (0, 1, 0)
  line L0 (810.6183, -461.2666) -> (810.6183, -397.2666) projected
  line L1 (836.2183, -461.2666) -> (836.2183, -397.2666) projected
  line L2 (353.8183, -461.2666) -> (353.8183, -397.2666) projected
  line L3 (328.2183, -397.2666) -> (328.2183, -461.2666) projected
  point P0 (0, 2598.7334)
  point P1 (823.4183, -446.6488)
  point P2 (341.0183, -446.6488)
  dimension "d138" = 12.8
  dimension "d139" = 12.8
  dimension "d140" = 12.8
  measures "d138" distance from line of point (823.418, -446.649) L1
  measures "d139" distance from line of L0 point (823.418, -446.649)
  measures "d140" distance from line of point (341.018, -446.649) L2
ref_plane "Work Plane37" through (1746.7139, 823.4183, -3045.3822) normal (0, 1, 0) x (-1, 0, 0)
sketch "Sketch46" plane through (1746.7139, 823.4183, -3045.3822) normal (0, 1, 0) x (-1, 0, 0)
  line L0 (-800, -744.2178) -> (-800, -674.6178) projected
  line L1 (3800, -744.2178) -> (3800, -674.6178) projected
  line L2 (-800, -744.2178) -> (3800, -744.2178) projected
  line L3 (-800, -750.6178) -> (3800, -750.6178) projected
  line L4 (0, 49.3822) -> (3000, 49.3822) projected
  line L5 (1500, -750.6178) -> (1500, 49.3822)
  line L6 (1487.2, 49.3822) -> (1487.2, -750.6178)
  line L7 (1500, -750.6178) -> (1487.2, -750.6178)
  point P0 (1746.7139, 3045.3822)
  dimension "d141" = 12.8
  dimension "d142" = 2300
  constraints: 6 end point, 3 perpendicular, 2 midpoint, 2 point on line
  measures "d141" distance between parallel lines of L6 L5
  measures "d142" distance between parallel lines of L0 L5
revolve "Revolution1" add sketch "Sketch46" angle 360 about axis through (246.7139, 823.4183, -3796) along (0, 0, 1) separate body
sketch "Sketch47" plane through (1746.7139, 823.4183, -3045.3822) normal (0, 1, 0) x (-1, 0, 0)
  line L0 (-800, -744.2178) -> (3800, -744.2178) projected
  line L1 (0, 49.3822) -> (3000, 49.3822) projected
  line L2 (100, -744.2178) -> (100, 49.3822)
  line L3 (87.2, 49.3822) -> (87.2, -744.2178)
  line L4 (100, -744.2178) -> (87.2, -744.2178)
  line L5 (-800, -744.2178) -> (-800, -674.6178) projected
  point P0 (1746.7139, 3045.3822)
  dimension "d144" = 12.8
  dimension "d145" = 900
  constraints: 6 end point, 4 point on line, 3 perpendicular
  measures "d144" distance between parallel lines of L3 L2
  measures "d145" distance between parallel lines of L5 L2
revolve "Revolution2" add sketch "Sketch47" angle 360 about axis through (1646.7139, 823.4183, -3789.6) along (0, 0, 1) separate body
sketch "Sketch48" plane through (1746.7139, 823.4183, -3045.3822) normal (0, 1, 0) x (-1, 0, 0)
  line L0 (0, 49.3822) -> (3000, 49.3822) projected
  line L1 (-800, -744.2178) -> (3800, -744.2178) projected
  line L2 (-800, -744.2178) -> (-800, -674.6178) projected
  line L3 (2912.8, 49.3822) -> (2912.8, -744.2178)
  line L4 (2900, -744.2178) -> (2900, 49.3822)
  line L5 (2900, 49.3822) -> (2912.8, 49.3822)
  line L6 (2912.8, -744.2178) -> (2900, -744.2178)
  line L7 (3000, -14.6178) -> (3000, 42.9822) projected
  point P0 (1746.7139, 3045.3822)
  dimension "d147" = 12.8
  dimension "d148" = 100
  constraints: 8 end point, 4 point on line, 3 perpendicular, 1 parallel
  measures "d147" distance between parallel lines of L3 L4
  measures "d148" distance between parallel lines of L4 L7
revolve "Revolution3" add sketch "Sketch48" angle 360 about axis through (-1153.2861, 823.4183, -3789.6) along (0, 0, 1) separate body
move or copy body "Move Body5" bodies to move or copy 11 copy no translate (40, 0, 0)
move or copy body "Move Body6" bodies to move or copy 17 copy no translate (40, 0, 0)
move or copy body "Move Body7" bodies to move or copy 13 copy no translate (40, 0, 0)
move or copy body "Move Body8" bodies to move or copy 15 copy no translate (40, 0, 0)
move or copy body "Move Body9" bodies to move or copy 16 copy no translate (40, 0, 0)
move or copy body "Move Body10" bodies to move or copy 12 copy no translate (40, 0, 0)
move or copy body "Move Body11" bodies to move or copy 14 copy no translate (40, 0, 0)
move or copy body "Move Body12" bodies to move or copy 16 copy no translate (40, 0, 0)
move or copy body "Move Body13" bodies to move or copy 15 copy no translate (40, 0, 0)
move or copy body "Move Body14" bodies to move or copy 17 copy no translate (40, 0, 0)
sketch "Sketch49" plane through (1746.7139, 823.4183, -3045.3822) normal (0, 1, 0) x (-1, 0, 0)
  line L0 (-840, -750.6178) -> (3760, -750.6178) projected
  line L1 (3760, -744.2178) -> (3760, -674.6178) projected
  line L2 (2832.8, -744.2178) -> (2832.8, 49.3822) projected
  line L3 (-40, 49.3822) -> (2960, 49.3822) projected
  line L4 (3555.5982, -692.4186) -> (2832.8, 49.3822)
  line L5 (2832.8, 49.3822) -> (2823.6324, 40.4494)
  line L6 (3555.5982, -710.7601) -> (3555.5982, -692.4186)
  line L7 (2823.6324, 40.4494) -> (3555.5982, -710.7601)
  line L8 (3555.5982, -710.7601) -> (3555.5982, -692.4186)
  point P0 (1746.7139, 3045.3822)
  dimension "d180" = 12.8
  constraints: 10 end point, 2 perpendicular, 1 collinear, 1 parallel
  measures "d180" distance between parallel lines of L7 L4
revolve "Revolution4" add sketch "Sketch49" angle 360 about axis through (-1076.9185, 823.4183, -3004.9328) along (-0.6978736, 0, -0.716221) separate body
sketch "Sketch50" plane through (1746.7139, 823.4183, -3045.3822) normal (0, 1, 0) x (-1, 0, 0)
  line L0 (-40, 49.3822) -> (2960, 49.3822) projected
  line L1 (-840, -744.2178) -> (3760, -744.2178) projected
  line L2 (2807.2, -744.2178) -> (2807.2, 49.3822) projected
  line L3 (1432.8, -750.6178) -> (1432.8, 49.3822) projected
  line L4 (2807.2, 49.3822) -> (2123.2963, -744.2178)
  line L5 (2123.2963, -744.2178) -> (2113.6, -735.8618)
  line L6 (2113.6, -735.8618) -> (2771.1777, 27.1895)
  line L7 (2780.874, 18.8336) -> (2771.1777, 27.1895)
  point P0 (1746.7139, 3045.3822)
  dimension "d182" = 12.8
  dimension "d183" = 693.6
  constraints: 8 end point, 3 perpendicular, 2 point on line
  measures "d182" distance between parallel lines of L4 L6
  measures "d183" distance from line of L5.end L2
revolve "Revolution5" add sketch "Sketch50" angle 360 about axis through (-366.8861, 823.4183, -3781.244) along (-0.6528114, 0, 0.7575205) separate body contours L4 L5 L6 L7
sketch "Sketch51" plane through (1746.7139, 823.4183, -3045.3822) normal (0, 1, 0) x (-1, 0, 0)
  line L0 (-840, -744.2178) -> (3760, -744.2178) projected
  line L1 (-40, 49.3822) -> (2960, 49.3822) projected
  line L2 (1432.8, -750.6178) -> (1432.8, 49.3822) projected
  line L3 (2761.4814, 35.5455) -> (2103.9037, -727.5058) projected
  line L4 (2103.9037, -727.5058) -> (1432.8, 49.3822)
  line L5 (1432.8, 49.3822) -> (1423.1136, 41.0148)
  line L6 (1423.1136, 41.0148) -> (2069.1575, -706.8633)
  line L7 (2069.1575, -706.8633) -> (2078.8439, -698.4959)
  point P0 (1746.7139, 3045.3822)
  dimension "d185" = 12.8
  constraints: 8 end point, 3 perpendicular, 1 point on line
  measures "d185" distance between parallel lines of L6 L4
revolve "Revolution6" add sketch "Sketch51" angle 360 about axis through (-357.1899, 823.4183, -3772.888) along (0.6537063, 0, 0.7567483) separate body
sketch "Sketch52" plane through (1746.7139, 823.4183, -3045.3822) normal (0, 1, 0) x (-1, 0, 0)
  line L0 (1407.2, -750.6178) -> (1407.2, 49.3822) projected
  line L1 (-840, -750.6178) -> (3760, -750.6178) projected
  line L2 (1407.2, 41.0143) -> (723.2859, -750.6178)
  line L3 (723.2859, -750.6178) -> (713.6, -742.2498)
  line L4 (713.6, -742.2498) -> (1397.5141, 49.3822)
  line L5 (1397.5141, 49.3822) -> (1407.2, 41.0143)
  line L6 (-40, 49.3822) -> (2960, 49.3822) projected
  point P0 (1746.7139, 3045.3822)
  dimension "d187" = 12.8
  dimension "d188" = 693.6
  constraints: 8 end point, 3 point on line, 2 perpendicular, 1 parallel
  measures "d187" distance between parallel lines of L4 L2
  measures "d188" distance from line of L0 L3.end
revolve "Revolution7" add sketch "Sketch52" angle 360 about axis through (1033.1139, 823.4183, -3787.632) along (-0.6537468, 0, 0.7567134) separate body contours L2 L3 L4 L5
sketch "Sketch53" plane through (1746.7139, 823.4183, -3045.3822) normal (0, 1, 0) x (-1, 0, 0)
  line L0 (1387.8281, 57.7502) -> (703.9141, -733.8819) projected
  line L1 (-40, 49.3822) -> (2960, 49.3822) projected
  line L2 (32.8, 49.3822) -> (32.8, -744.2178) projected
  line L3 (749.9555, -680.5888) -> (32.8, 31.3461)
  line L4 (32.8, 49.3822) -> (758.9733, -671.5048)
  line L5 (758.9733, -671.5048) -> (749.9555, -680.5888)
  point P0 (1746.7139, 3045.3822)
  dimension "d190" = 12.8
  constraints: 6 end point, 2 point on line, 1 parallel, 1 perpendicular
  measures "d190" distance between parallel lines of L3 L4
revolve "Revolution8" add sketch "Sketch53" angle 360 about axis through (996.7584, 823.4183, -3725.971) along (0.7096852, 0, 0.7045189) separate body contours L4 L5 L0 | L0 L3 L2 L4
sketch "Sketch54" plane through (1746.7139, 823.4183, -3045.3822) normal (0, 1, 0) x (-1, 0, 0)
  line L0 (20.1944, 48.0325) -> (-647.9141, -691.6592)
  line L1 (-647.9141, -691.6592) -> (-638.4152, -700.2389)
  line L2 (-638.4152, -700.2389) -> (29.6933, 39.4528)
  line L3 (29.6933, 39.4528) -> (20.1944, 48.0325)
  point P0 (1746.7139, 3045.3822)
  dimension "d192" = 12.8
  constraints: 8 end point, 2 parallel, 1 perpendicular
  measures "d192" distance between parallel lines of L0 L2
revolve "Revolution9" add sketch "Sketch54" angle 360 about axis through (2385.1291, 823.4183, -3745.6211) along (-0.6702862, 0, 0.7421027) separate body
ref_plane "Work Plane38" through (1746.7139, 341.0183, -3045.3822) normal (0, 1, 0) x (-1, 0, 0)
sketch "Sketch55" plane through (1746.7139, 341.0183, -3045.3822) normal (0, 1, 0) x (-1, 0, 0)
  line L0 (-628.9163, -708.8185) -> (39.1922, 30.8731) projected
  line L1 (-628.9163, -708.8185) -> (39.1922, 30.8731)
  line L2 (39.1922, 30.8731) -> (29.6933, 39.4528)
  line L3 (29.6933, 39.4528) -> (-646.1646, -708.8185)
  line L4 (-646.1646, -708.8185) -> (-628.9163, -708.8185)
  point P0 (1746.7139, 3045.3822)
  dimension "d194" = 12.8
  constraints: 8 end point, 1 collinear, 1 horizontal, 1 parallel, 1 perpendicular
  measures "d194" distance between parallel lines of L1 L3
revolve "Revolution10" add sketch "Sketch55" angle 360 about axis through (1717.0206, 341.0183, -3005.9294) along (0.6702862, 0, -0.7421027) separate body
sketch "Sketch56" plane through (1746.7139, 341.0183, -3045.3822) normal (0, 1, 0) x (-1, 0, 0)
  line L0 (32.8, 49.3822) -> (32.8, -744.2178) projected
  line L1 (32.8, -744.2178) -> (32.8, 49.3822)
  line L2 (32.8, 49.3822) -> (20, 49.3822)
  line L3 (20, 49.3822) -> (20, -744.2178)
  line L4 (20, -744.2178) -> (32.8, -744.2178)
  point P0 (1746.7139, 3045.3822)
  dimension "d196" = 12.8
  constraints: 8 end point, 3 perpendicular, 1 collinear
  measures "d196" distance between parallel lines of L1 L3
revolve "Revolution11" add sketch "Sketch56" angle 360 about axis through (1726.7139, 341.0183, -2996) along (0, 0, -1) separate body
sketch "Sketch57" plane through (1746.7139, 341.0183, -3045.3822) normal (0, 1, 0) x (-1, 0, 0)
  line L0 (32.8, 49.3822) -> (758.9733, -671.5048) projected
  line L1 (32.8, 49.3822) -> (786.0886, -698.4227)
  line L2 (786.0886, -698.4227) -> (777.0707, -707.5067)
  line L3 (777.0707, -707.5067) -> (50.8974, 13.3804)
  line L4 (59.9152, 22.4644) -> (50.8974, 13.3804)
  point P0 (1746.7139, 3045.3822)
  dimension "d198" = 12.8
  constraints: 8 end point, 3 perpendicular, 2 point on line
  measures "d198" distance between parallel lines of L1 L3
revolve "Revolution12" add sketch "Sketch57" angle 360 about axis through (969.6432, 341.0183, -3752.8889) along (0.7096852, 0, 0.7045189) separate body
sketch "Sketch58" plane through (1746.7139, 341.0183, -3045.3822) normal (0, 1, 0) x (-1, 0, 0)
  line L0 (1387.8281, 57.7502) -> (703.9141, -733.8819) projected
  line L1 (703.9141, -733.8819) -> (1373.0719, 40.6698)
  line L2 (1373.0719, 40.6698) -> (1382.7578, 32.3018)
  line L3 (1382.7578, 32.3018) -> (713.6, -742.2498)
  line L4 (703.9141, -733.8819) -> (713.6, -742.2498)
  point P0 (1746.7139, 3045.3822)
  dimension "d200" = 12.8
  constraints: 8 end point, 3 perpendicular, 1 point on line
  measures "d200" distance between parallel lines of L3 L1
revolve "Revolution13" add sketch "Sketch58" angle 360 about axis through (363.9561, 341.0183, -3013.0804) along (0.6537468, 0, -0.7567134) separate body
sketch "Sketch59" plane through (1746.7139, 341.0183, -3045.3822) normal (0, 1, 0) x (-1, 0, 0)
  line L0 (1407.2, -750.6178) -> (1407.2, 49.3822) projected
  line L1 (1407.2, 49.3822) -> (1407.2, -750.6178)
  line L2 (1407.2, -750.6178) -> (1420, -750.6178)
  line L3 (1420, -750.6178) -> (1420, 49.3822)
  line L4 (1420, 49.3822) -> (1407.2, 49.3822)
  line L5 (1407.2, -750.6178) -> (1420, -750.6178)
  point P0 (1746.7139, 3045.3822)
  dimension "d202" = 12.8
  constraints: 10 end point, 3 perpendicular, 2 equal length
  measures "d202" distance between parallel lines of L3 L1
revolve "Revolution14" add sketch "Sketch59" angle 360 about axis through (326.7139, 341.0183, -3796) along (0, 0, 1) separate body
sketch "Sketch60" plane through (1746.7139, 341.0183, -3045.3822) normal (0, 1, 0) x (-1, 0, 0)
  line L0 (2088.5303, -690.1284) -> (1442.4864, 57.7497) projected
  line L1 (1457.7474, 40.0831) -> (2114.7248, -720.4519)
  line L2 (2114.7248, -720.4519) -> (2105.0384, -728.8193)
  line L3 (2114.7248, -720.4519) -> (2105.0384, -728.8193)
  line L4 (2105.0384, -728.8193) -> (1442.4864, 38.169)
  line L5 (1442.4864, 38.169) -> (1442.4864, 57.7497)
  point P0 (1746.7139, 3045.3822)
  dimension "d204" = 12.8
  constraints: 10 end point, 2 collinear, 2 perpendicular, 1 point on line, 1 vertical
  measures "d204" distance between parallel lines of L4 L1
revolve "Revolution15" add sketch "Sketch60" angle 360 about axis through (-358.3245, 341.0183, -3774.2016) along (0.6537063, 0, 0.7567483) separate body
sketch "Sketch61" plane through (1746.7139, 341.0183, -3045.3822) normal (0, 1, 0) x (-1, 0, 0)
  line L0 (2761.4814, 35.5455) -> (2103.9037, -727.5058) projected
  line L1 (2103.9037, -727.5058) -> (2761.4814, 35.5455)
  line L2 (2761.4814, 35.5455) -> (2771.1777, 27.1895)
  line L3 (2771.1777, 27.1895) -> (2113.6, -735.8618)
  line L4 (2113.6, -735.8618) -> (2103.9037, -727.5058)
  point P0 (1746.7139, 3045.3822)
  dimension "d206" = 12.8
  constraints: 8 end point, 2 equal length, 2 perpendicular
  measures "d206" distance between parallel lines of L3 L1
revolve "Revolution16" add sketch "Sketch61" angle 360 about axis through (-1024.4638, 341.0183, -3018.1927) along (0.6528114, 0, -0.7575205) separate body
sketch "Sketch62" plane through (1746.7139, 341.0183, -3045.3822) normal (0, 1, 0) x (-1, 0, 0)
  line L0 (2807.2, -744.2178) -> (2807.2, 49.3822) projected
  line L1 (2807.2, 49.3822) -> (2807.2, -744.2178)
  line L2 (2807.2, -744.2178) -> (2822.7011, -744.2178)
  line L3 (2822.7011, -744.2178) -> (2822.7011, 49.3822)
  line L4 (2822.7011, 49.3822) -> (2807.2, 49.3822)
  point P0 (1746.7139, 3045.3822)
  constraints: 8 end point, 3 perpendicular, 1 collinear
revolve "Revolution17" add sketch "Sketch62" angle 360 about axis through (-1075.9872, 341.0183, -3789.6) along (0, 0, 1) separate body